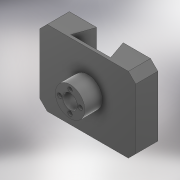
# Autodesk Inventor part: 1
Saved by Autodesk Inventor 2022 (Build 260153000, 153)
## iProperties
Company: HS Emden/Leer
Created: 2023-07-21
Part Number: 1
Material: PMMA-Kunststoff
Document SubType Name: Modeling
Designer: Yaman Alsaady
Density: 1.188 g/cm^3
Appearance: Glatt - Schwarz
Project: Delta-Robot
Author: Yaman Alsaady
Title: Holder
## iProperties of the stored document _3D-Druck.ipt
Created: 2023-08-01
Part Number: _3D-Druck
Material: Generisch
Document SubType Name: Modeling
Designer: Alsaady
Density: 1 g/cm^3
Appearance: Vorgabe
Author: Alsaady
Autodesk Inventor part; units mm, degrees
ref_plane "YZ Plane" through (0, 0, 0) normal (1, 0, 0) x (0, 1, 0)
ref_plane "XZ Plane" through (0, 0, 0) normal (0, 1, 0) x (-1, 0, 0)
ref_plane "XY Plane" through (0, 0, 0) normal (0, 0, 1) x (1, 0, 0)
sketch "Skizze1" plane through (0, 0, 0) normal (0, 0, 1) x (1, 0, 0)
  line L0 (-32.5, 25.5) -> (32.5, 25.5)
  line L1 (32.5, 25.5) -> (32.5, -25.5)
  line L2 (32.5, -25.5) -> (-32.5, -25.5)
  line L3 (-32.5, -25.5) -> (-32.5, 25.5)
  line L4 (0, -35.7) -> (0, 35.7) projected
  line L5 (-45.5, 0) -> (45.5, 0) projected
  point P0 (0, 0)
  point P1 (0, 25.5)
  point P2 (32.5, 0)
  dimension "d0" = 51
  dimension "d1" = 65
  constraints: 8 end point, 2 midpoint, 2 parallel, 2 point on line, 1 horizontal, 1 perpendicular
  measures "d0" distance of L0.end L1.end
  measures "d1" distance of L0.start L0.end
extrude "Extrusion1" add sketch "Skizze1" along normal blind 15
sketch "Skizze2" plane through (-32.5, -25.5, 0) normal (0, -1, 0) x (1, 0, 0)
  line L0 (23.5, 0) -> (41.5, 0)
  line L1 (41.5, 0) -> (46, 13)
  line L2 (46, 13) -> (19, 13)
  line L3 (19, 13) -> (23.5, 0)
  line L4 (0, 0) -> (65, 0) projected
  line L5 (0, 15) -> (65, 15) construction
  circle A0 centre (32.5, 6.5) radius 2.15
  line L6 (32.5, 0) -> (32.5, 13) construction
  point P0 (32.5, 0)
  point P1 (32.5, 6.5)
  dimension "d4" = 18
  dimension "d5" = 27
  dimension "d6" = 13
  dimension "d20" = 4.3
  constraints: 10 end point, 4 midpoint, 1 centre point, 1 coincident, 1 horizontal, 1 parallel, 1 perpendicular
  measures "d4" distance of L0.start L0.end
  measures "d5" distance of L1.end L2.end
  measures "d6" distance from line of L2 L0.end
  measures "d20" diameter of A0
extrude "Extrusion2" cut sketch "Skizze2" against normal through all contours L3 L2 L1 L0 | A0
extrude "Extrusion5" add sketch "Skizze2" against normal blind 9
chamfer "Fase1" distance 5 angle 45 4 edges at (-32.5, 25.5, 7.5) (32.5, 25.5, 7.5) (32.5, -25.5, 7.5) (-32.5, -25.5, 7.5)
sketch "Skizze3" plane through (0, 0, 15) normal (0, 0, 1) x (1, 0, 0)
  circle A0 centre (0, 0) radius 10
  dimension "d12" = 20
  constraints: 1 centre point, 1 coincident
  measures "d12" diameter of A0
extrude "Extrusion3" add sketch "Skizze3" along normal blind 12
sketch "Skizze4" plane through (0, 0, 27) normal (0, 0, 1) x (1, 0, 0)
  circle A0 centre (0, 0) radius 5
  dimension "d15" = 10
  constraints: 1 centre point, 1 coincident
  measures "d15" diameter of A0
extrude "Extrusion4" cut sketch "Skizze4" against normal through all
sketch "Skizze5" plane through (0, 0, 27) normal (0, 0, 1) x (1, 0, 0)
  circle A0 centre (7, 0) radius 1.5
  line L0 (-45.5, 0) -> (45.5, 0) projected
  circle A1 centre (0, 0) radius 5 projected
  circle A2 centre (0, 0) radius 10 projected
  circle A3 centre (0, 7) radius 1.5
  circle A4 centre (-7, 0) radius 1.5
  circle A5 centre (0, -7) radius 1.5
  dimension "d21" = 3
  dimension "d22" = 7
  dimension "d25" = 360
  constraints: 4 centre point, 1 point on line, 9 other
  measures "d21" diameter of A0
  measures "d22" distance of point (0, 0) A0.centre
extrude "Extrusion6" cut sketch "Skizze5" against normal through all contours L0 A0 | A0 L0 | A4 L0 | L0 A4 | A3 | A5
sketch "Skizze6" plane through (0, 0, 27) normal (0, 0, 1) x (1, 0, 0)
  line L0 (15.25, -15.25) -> (-15.25, -15.25)
  line L1 (-15.25, -15.25) -> (-15.25, 15.25)
  line L2 (-15.25, 15.25) -> (15.25, 15.25)
  line L3 (15.25, 15.25) -> (15.25, -15.25)
  line L4 (15.25, -15.25) -> (-15.25, 15.25) construction
  line L5 (-15.25, -15.25) -> (15.25, 15.25) construction
  circle A0 centre (15.25, 15.25) radius 2
  circle A1 centre (-15.25, 15.25) radius 2
  circle A2 centre (-15.25, -15.25) radius 2
  circle A3 centre (15.25, -15.25) radius 2
  point P0 (0, 0)
  dimension "d29" = 30.5
  dimension "d30" = 4
  constraints: 12 end point, 4 centre point, 4 coincident, 3 equal radius, 2 midpoint, 2 parallel, 2 perpendicular, 1 horizontal
  measures "d29" distance of L1.end L2.end
  measures "d30" diameter of A0
extrude "Extrusion7" [suppressed]
